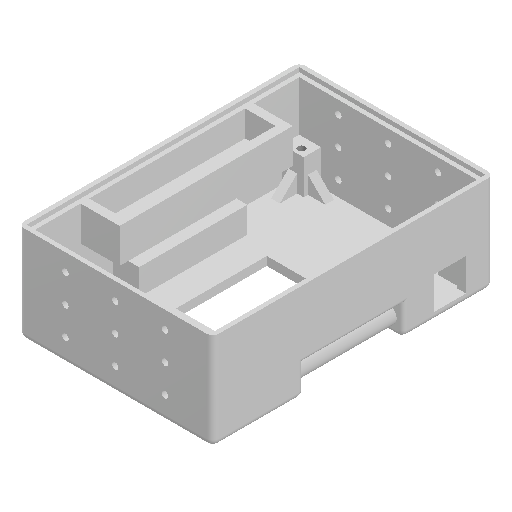
# Autodesk Inventor part: Base
Saved by Autodesk Inventor 2025.2 (Build 292293000, 293)
## iProperties
Created: 2025-10-17
Part Number: Base
Material: ABS Plastic
Document SubType Name: Modeling
Designer: Ricardo
Density: 1.06 g/cm^3
Appearance: Smooth - White
Author: Ricardo
Autodesk Inventor part; units mm, degrees
ref_plane "YZ Plane" through (0, 0, 0) normal (1, 0, 0) x (0, 1, 0)
ref_plane "XZ Plane" through (0, 0, 0) normal (0, 1, 0) x (-1, 0, 0)
ref_plane "XY Plane" through (0, 0, 0) normal (0, 0, 1) x (1, 0, 0)
sketch "Sketch1" plane through (0, 0, 0) normal (0, 1, 0) x (-1, 0, 0)
  line L0 (0, 0) -> (45, 0)
  line L1 (45, 0) -> (45, -65)
  line L2 (45, -65) -> (0, -65)
  line L3 (0, -65) -> (0, 0)
  dimension "d0" = 45
  dimension "d1" = 65
  constraints: 8 end point, 2 parallel, 1 horizontal, 1 perpendicular
  measures "d0" distance of L1.end L2.end
  measures "d1" distance of L0.end L1.end
extrude "Extrusion1" add sketch "Sketch1" against normal blind 3.5
sketch "Sketch2" plane through (0, 0, 0) normal (0, 1, 0) x (1, 0, 0)
  line L0 (-43, 2) -> (-2, 2)
  line L1 (-2, 2) -> (-2, 63)
  line L2 (-2, 63) -> (-43, 63)
  line L3 (-43, 63) -> (-43, 2)
  line L4 (0, 65) -> (-45, 65) projected
  line L5 (-45, 65) -> (-45, 0) projected
  line L6 (-45, 0) -> (0, 0) projected
  line L7 (0, 0) -> (0, 65) projected
  dimension "d4" = 2
  dimension "d5" = 2
  dimension "d6" = 2
  dimension "d7" = 2
  constraints: 8 end point, 2 parallel, 1 horizontal, 1 perpendicular
  measures "d4" distance between parallel lines of L5 L3
  measures "d5" distance between parallel lines of L4 L2
  measures "d6" distance between parallel lines of L7 L1
  measures "d7" distance between parallel lines of L6 L0
extrude "Extrusion2" cut sketch "Sketch2" against normal blind 1.5 contours L3 L2 L1 L0
sketch "Sketch3" plane through (0, -1.5, 0) normal (0, 1, 0) x (1, 0, 0)
  line L0 (-2, 63) -> (-2, 2) projected
  line L1 (-43, 63) -> (-2, 63) projected
  line L2 (-43, 2) -> (-43, 63) projected
  line L3 (-2, 2) -> (-43, 2) projected
  line L4 (-45, 0) -> (0, 0) projected
  line L5 (0, 65) -> (-45, 65) projected
  line L6 (0, 0) -> (0, 65) projected
  line L7 (-45, 65) -> (-45, 0) projected
  line L8 (-30.5, 22) -> (-14.5, 22)
  line L9 (-14.5, 22) -> (-14.5, 43)
  line L10 (-14.5, 43) -> (-30.5, 43)
  line L11 (-30.5, 43) -> (-30.5, 22)
  line L12 (-43, 2) -> (-43, 63) projected
  line L13 (-22.5, 0) -> (-22.5, 65) construction
  line L14 (0, 32.5) -> (-45, 32.5) construction
  dimension "d10" = 16
  dimension "d11" = 21
  constraints: 12 end point, 4 midpoint, 3 parallel, 1 horizontal, 1 perpendicular, 2 other
  measures "d10" distance of L10.end L9.end
  measures "d11" distance of L10.end L8.start
extrude "Extrusion3" cut sketch "Sketch3" against normal blind 3 contours L11 L10 L9 L8
sketch "Sketch4" plane through (0, -1.5, 0) normal (0, 1, 0) x (1, 0, 0)
  line L0 (-30.5, 22) -> (-30.5, 43) construction
  line L1 (-14.5, 43) -> (-14.5, 22) construction
  line L2 (-14.5, 32.5) -> (-30.5, 32.5) construction
  line L3 (-45, 65) -> (0, 65) construction
  line L4 (-22.5, 65) -> (-22.5, 5) construction
  circle A0 centre (-22.5, 12) radius 5.25
  circle A1 centre (-22.5, 12) radius 6
  line L5 (-45, 0) -> (0, 0) projected
  line L6 (-22.5, 12) -> (-30.82, 16.8036) construction
  line L7 (-22.5, 12) -> (-31.5933, 6.75) construction
  line L8 (-27.0466, 14.625) -> (-27.8953, 14.625)
  line L9 (-27.0466, 9.375) -> (-27.8953, 9.375)
  point P0 (-28.3926, 10.8696)
  point P1 (-27.637, 10.9167)
  dimension "d14" = 10.5
  dimension "d15" = 12
  dimension "d181" = 12
  dimension "d200" = 60
  dimension "d201" = 60
  constraints: 12 end point, 6 point on circle, 4 midpoint, 2 centre point, 2 point on line, 1 coincident, 1 horizontal, 1 parallel, 1 vertical
  measures "d14" diameter of A0
  measures "d15" diameter of A1
  measures "d181" distance from line of L5 A0.centre
  measures "d200" angle of L4 L7
  measures "d201" angle of L6 L4
sketch "Sketch6" plane through (0, -1.5, 0) normal (0, 1, 0) x (1, 0, 0)
  line L0 (-14.5, 43) -> (-30.5, 43) projected
  line L1 (-30.5, 43) -> (-30.5, 22) projected
  line L2 (-30.5, 22) -> (-14.5, 22) projected
  line L3 (-14.5, 22) -> (-14.5, 43) projected
  line L4 (-2, 63) -> (-43, 63) projected
  line L5 (-43, 63) -> (-43, 2) projected
  line L6 (-43, 2) -> (-2, 2) projected
  line L7 (-2, 2) -> (-2, 63) projected
  line L8 (-45, 0) -> (-45, 65) projected
  line L9 (-45, 65) -> (0, 65) projected
  line L10 (0, 65) -> (0, 0) projected
  line L11 (0, 0) -> (-45, 0) projected
  line L12 (-43, 2) -> (-43, 63) projected
  line L13 (-43, 63) -> (-38, 63)
  line L14 (-38, 63) -> (-38, 59)
  line L15 (-38, 59) -> (-43, 59)
  line L16 (-43, 59) -> (-43, 63)
  line L17 (-43, 63) -> (-2, 63) projected
  line L18 (-2, 63) -> (-7, 63)
  line L19 (-7, 63) -> (-7, 59)
  line L20 (-7, 59) -> (-2, 59)
  line L21 (-2, 59) -> (-2, 63)
  line L22 (-43, 2) -> (-38, 2)
  line L23 (-38, 2) -> (-38, 6)
  line L24 (-38, 6) -> (-43, 6)
  line L25 (-43, 6) -> (-43, 2)
  line L26 (-2, 2) -> (-7, 2)
  line L27 (-7, 2) -> (-7, 6)
  line L28 (-7, 6) -> (-2, 6)
  line L29 (-2, 6) -> (-2, 2)
  point P0 (-43, 59)
  point P1 (-2, 59)
  point P2 (-2, 6)
  dimension "d30" = 5
  dimension "d31" = 4
  dimension "d32" = 5
  dimension "d33" = 4
  dimension "d34" = 5
  dimension "d35" = 4
  dimension "d36" = 5
  dimension "d37" = 4
  constraints: 32 end point, 8 parallel, 4 horizontal, 4 perpendicular
  measures "d30" distance of L14.end L15.end
  measures "d31" distance of L13.end L14.end
  measures "d32" distance of L20.end L19.end
  measures "d33" distance of L18.end L19.end
  measures "d34" distance of L24.end L23.end
  measures "d35" distance of L22.end L23.end
  measures "d36" distance of L27.end L28.end
  measures "d37" distance of L26.end L27.end
extrude "Extrusion6" add sketch "Sketch6" along normal blind 8 contours L7 L20 L19 L4 | L14 L15 L5 L4 | L7 L6 L27 L28 | L24 L23 L6 L5
sketch "Sketch7" plane through (0, 6.5, 0) normal (0, 1, 0) x (1, 0, 0)
  line L0 (-2, 63) -> (-2, 59) projected
  line L1 (-2, 59) -> (-7, 59) projected
  line L2 (-7, 59) -> (-7, 63) projected
  line L3 (-7, 63) -> (-2, 63) projected
  line L4 (-7, 6) -> (-2, 6) projected
  line L5 (-2, 6) -> (-2, 2) projected
  line L6 (-2, 2) -> (-7, 2) projected
  line L7 (-7, 2) -> (-7, 6) projected
  line L8 (-38, 59) -> (-43, 59) projected
  line L9 (-43, 59) -> (-43, 63) projected
  line L10 (-43, 63) -> (-38, 63) projected
  line L11 (-38, 63) -> (-38, 59) projected
  line L12 (-43, 2) -> (-43, 6) projected
  line L13 (-43, 6) -> (-38, 6) projected
  line L14 (-38, 6) -> (-38, 2) projected
  line L15 (-38, 2) -> (-43, 2) projected
  line L16 (-43, 4) -> (-40, 4) construction
  line L17 (-39.4871, 2) -> (-39.4871, 4.5) construction
  line L18 (-43, 6) -> (-43, 59) projected
  line L19 (-2, 59) -> (-2, 6) projected
  line L20 (0, 0) -> (-45, 0) construction
  line L21 (-22.5, 0) -> (-22.5, 65) construction
  line L22 (-45, 65) -> (0, 65) construction
  point P0 (-5, 60.5)
  point P1 (-5, 4.5)
  point P2 (-40, 60.5)
  dimension "d49" = 3
  dimension "d50" = 2.5
  dimension "d51" = 3
  dimension "d52" = 2.5
  dimension "d53" = 3
  dimension "d54" = 2.5
  dimension "d55" = 2.5
  dimension "d56" = 3
  constraints: 6 end point, 3 midpoint, 1 coincident, 1 horizontal, 1 perpendicular, 1 point on line
  measures "d49" distance of L16.start L16.end
  measures "d50" distance of L17.start L17.end
  measures "d51" distance from line of L5 point (-5, 4.5)
  measures "d52" distance from line of L6 point (-5, 4.5)
  measures "d53" distance from line of L19 point (-5, 60.5)
  measures "d54" distance from line of L3 point (-5, 60.5)
  measures "d55" distance from line of L10 point (-40, 60.5)
  measures "d56" distance from line of L9 point (-40, 60.5)
hole "Hole1" at (-5, 6.5, -60.5) at (-5, 6.5, -4.5) at (-39.4871, 6.5, -4.5) at (-40, 6.5, -60.5) direction (0, -1, 0) diameter 1.7294 depth 3 tip angle 118 thread size "M2x0.25" class "6H" standard "ISO Metric profile"
sketch "Sketch8" plane through (0, 0, 0) normal (0, 1, 0) x (1, 0, 0)
  line L0 (-43, 2) -> (-43, 6) projected
  line L1 (-43, 6) -> (-38, 6) projected
  line L2 (-38, 6) -> (-38, 2) projected
  line L3 (-38, 2) -> (-43, 2) projected
  line L4 (-43, 59) -> (-43, 6) projected
  line L5 (-43, 59) -> (-43, 63) projected
  line L6 (-43, 63) -> (-38, 63) projected
  line L7 (-38, 63) -> (-38, 59) projected
  line L8 (-38, 2) -> (-7, 2) projected
  line L9 (-2, 2) -> (-7, 2) projected
  line L10 (-2, 6) -> (-2, 2) projected
  line L11 (-7, 6) -> (-2, 6) projected
  line L12 (-7, 2) -> (-7, 6) projected
  line L13 (-7, 63) -> (-38, 63) projected
  line L14 (-7, 63) -> (-2, 63) projected
  line L15 (-2, 63) -> (-2, 59) projected
  line L16 (-2, 59) -> (-7, 59) projected
  line L17 (-7, 59) -> (-7, 63) projected
  line L18 (-2, 6) -> (-2, 59) projected
  line L19 (-45, 0) -> (-45, 65) projected
  line L20 (-45, 65) -> (0, 65) projected
  line L21 (0, 65) -> (0, 0) projected
  line L22 (0, 0) -> (-45, 0) projected
  line L23 (-45, 0) -> (0, 0)
  line L24 (0, 0) -> (0, 65)
  line L25 (0, 65) -> (-45, 65)
  line L26 (-45, 65) -> (-45, 0)
  line L27 (-2, 63) -> (-43, 63)
  line L28 (-43, 63) -> (-43, 2)
  line L29 (-43, 2) -> (-2, 2)
  line L30 (-2, 2) -> (-2, 63)
  line L31 (-43, 6) -> (-43, 59) projected
  line L32 (-45, 65) -> (-45, 0) projected
  line L33 (0, 65) -> (-45, 65) projected
  line L34 (-38, 63) -> (-7, 63) projected
  line L35 (-38, 63) -> (-43, 63) projected
  line L36 (0, 0) -> (0, 65) projected
  line L37 (-2, 59) -> (-2, 6) projected
  line L38 (-7, 2) -> (-38, 2) projected
  line L39 (-45, 0) -> (0, 0) projected
  line L40 (-43, 2) -> (-2, 2)
  line L41 (-2, 2) -> (-2, 63)
  line L42 (-2, 63) -> (-43, 63)
  line L43 (-43, 63) -> (-43, 2)
  line L44 (0, 0) -> (-45, 0)
  line L45 (-45, 0) -> (-45, 65)
  line L46 (-45, 65) -> (0, 65)
  line L47 (0, 65) -> (0, 0)
  line L48 (-38, 59) -> (-43, 59) projected
  point P0 (-38.13, 58.5)
  point P1 (-37.5, 3.3857)
  point P2 (-38.5896, 4.5)
  point P3 (-5.5, 3.3968)
  point P4 (-4.3968, 4.5)
  point P5 (-39.1545, 59)
  point P6 (-38, 5.2834)
  point P7 (-38, 59.903)
  point P8 (-2.7165, 59)
  constraints: 32 end point, 8 parallel, 4 horizontal, 4 perpendicular
extrude "Extrusion7" add sketch "Sketch8" along normal blind 18
sketch "Sketch9" plane through (0, 18, 0) normal (0, 1, 0) x (1, 0, 0)
  line L0 (-45, 65) -> (-45, 0) projected
  line L1 (-45, 0) -> (0, 0) projected
  line L2 (0, 0) -> (0, 65) projected
  line L3 (0, 65) -> (-45, 65) projected
  line L4 (-1, 1) -> (-44, 1)
  line L5 (-44, 1) -> (-44, 64)
  line L6 (-44, 64) -> (-1, 64)
  line L7 (-1, 64) -> (-1, 1)
  line L8 (-45, 0) -> (0, 0)
  line L9 (0, 0) -> (0, 65)
  line L10 (0, 65) -> (-45, 65)
  line L11 (-45, 65) -> (-45, 0)
  line L12 (0, 0) -> (-45, 0)
  line L13 (0, 65) -> (0, 0) projected
  line L14 (0, 0) -> (-45, 0) projected
  line L15 (-45, 0) -> (-45, 65) projected
  line L16 (-45, 65) -> (0, 65) projected
  line L17 (-2, 2) -> (-2, 63) projected
  line L18 (-2, 63) -> (-43, 63) projected
  line L19 (-43, 63) -> (-43, 2) projected
  line L20 (-43, 2) -> (-2, 2) projected
  line L21 (-45, 0) -> (0, 0)
  line L22 (0, 0) -> (0, 65)
  line L23 (0, 65) -> (-45, 65)
  line L24 (-45, 65) -> (-45, 0)
  dimension "d57" = 1
  dimension "d58" = 1
  dimension "d59" = 1
  dimension "d60" = 1
  constraints: 26 end point, 7 equal length, 3 horizontal, 3 perpendicular
  measures "d57" distance between parallel lines of L3 L6
  measures "d58" distance between parallel lines of L0 L5
  measures "d59" distance between parallel lines of L1 L4
  measures "d60" distance between parallel lines of L2 L7
extrude "Extrusion8" add sketch "Sketch9" along normal blind 1 contours L3 L2 L1 L0
fillet "Fillet3" radius 1.5 1 edges at (-22.5, -3.5, 0)
fillet "Fillet4" radius 1.5 1 edges at (-22.5, -3.5, -65)
sketch "Sketch10" plane through (-45, 19, -65) normal (-1, 0, 0) x (0, 0, 1)
  line L0 (18, -15.5) -> (12, -15.5) construction
  line L1 (18, -14) -> (12, -14)
  line L2 (12, -17) -> (18, -17)
  arc A0 (18, -17) -> (18, -14) centre (18, -15.5) ccw
  arc A1 (12, -14) -> (12, -17) centre (12, -15.5) ccw
  line L3 (63.5, -22.5) -> (1.5, -22.5) projected
  line L4 (0, -21) -> (0, 0) projected
  point P0 (65, -19)
  point P1 (15, -15.5)
  point P2 (0, -9.5)
  point P3 (0, -6.5)
  dimension "d65" = 6
  dimension "d66" = 3
  dimension "d67" = 5.5
  dimension "d71" = 15
  constraints: 8 end point, 4 point on circle, 4 tangent, 2 centre point, 1 horizontal, 1 midpoint, 1 parallel
  measures "d65" distance of L0.start L0.end
  measures "d66" diameter of A1
  measures "d67" distance between parallel lines of L3 L2
  measures "d71" distance from line of L4 point (15, -15.5)
extrude "Extrusion9" cut sketch "Sketch10" against normal blind 10
sketch "Sketch13" plane through (0, 19, 0) normal (1, 0, 0) x (0, 0, -1)
  line L0 (59, -20.5) -> (6, -20.5) projected
  line L1 (59, -20.5) -> (63, -20.5) projected
  line L2 (63, -20.5) -> (63, -12.5) projected
  line L3 (51, -13) -> (58.5, -13)
  line L4 (58.5, -13) -> (58.5, -20.5)
  line L5 (58.5, -20.5) -> (51, -20.5)
  line L6 (51, -20.5) -> (51, -13)
  line L7 (51, -16.75) -> (58.5, -16.75) construction
  line L8 (54.75, -20.5) -> (54.75, -13) construction
  line L9 (65, 0) -> (65, -21) construction
  point P0 (0, -19)
  dimension "d82" = 7.5
  dimension "d83" = 7.5
  dimension "d84" = 0
  dimension "d86" = 6.5
  constraints: 12 end point, 4 midpoint, 2 parallel, 1 horizontal, 1 perpendicular
  measures "d82" distance of L4.end L5.end
  measures "d83" distance of L3.end L4.end
  measures "d84" distance between parallel lines of L0 L5
  measures "d86" distance between parallel lines of L9 L4
extrude "Extrusion11" cut sketch "Sketch13" against normal blind 10
sketch "Sketch17" plane through (0, -1.5, 0) normal (0, 1, 0) x (1, 0, 0)
  line L0 (-8, 45) -> (0, 45)
  line L1 (0, 45) -> (0, 20)
  line L2 (0, 20) -> (-8, 20)
  line L3 (-8, 20) -> (-8, 45)
  line L4 (0, 65) -> (-45, 65) projected
  line L5 (0, 0) -> (0, 65) projected
  line L6 (-22.5, 65) -> (-22.5, 0) construction
  line L7 (0, 0) -> (-45, 0) construction
  line L8 (-37, 45) -> (-45, 45)
  line L9 (-45, 45) -> (-45, 20)
  line L10 (-45, 20) -> (-37, 20)
  line L11 (-37, 20) -> (-37, 45)
  dimension "d104" = 8
  dimension "d105" = 25
  dimension "d106" = 20
  dimension "d107" = 0
  constraints: 18 end point, 4 symmetric about line, 2 midpoint, 2 parallel, 1 horizontal, 1 perpendicular
  measures "d104" distance of L1.end L2.end
  measures "d105" distance of L2.end L0.start
  measures "d106" distance from line of L4 L0.start
  measures "d107" distance between parallel lines of L5 L1
extrude "Extrusion16" add sketch "Sketch17" along normal blind 6
sketch "Sketch19" plane through (-45, 19, -65) normal (-1, 0, 0) x (0, 0, 1)
  arc A0 (18, -17) -> (18, -14) centre (18, -15.5) ccw projected
  line L0 (18, -14) -> (12, -14) projected
  arc A1 (12, -14) -> (12, -17) centre (12, -15.5) ccw projected
  line L1 (12, -17) -> (18, -17) projected
  arc A2 (0, -21) -> (1.5, -22.5) centre (1.5, -21) ccw projected
  line L2 (0, -21) -> (0, 0) projected
  line L3 (0, 0) -> (65, 0) projected
  line L4 (65, 0) -> (65, -21) projected
  arc A3 (63.5, -22.5) -> (65, -21) centre (63.5, -21) ccw projected
  line L5 (63.5, -22.5) -> (1.5, -22.5) projected
  line L6 (45, -14.5) -> (20, -14.5) projected
  line L7 (20, -14.5) -> (20, -20.5) projected
  line L8 (45, -20.5) -> (45, -14.5) projected
  line L9 (21, -22.5) -> (44, -22.5)
  line L10 (44, -22.5) -> (44, -15.5)
  line L11 (44, -15.5) -> (21, -15.5)
  line L12 (21, -15.5) -> (21, -22.5)
  point P0 (65, -19)
  point P1 (19.5, -7.5)
  point P2 (21, -19)
  point P3 (44, -22.5)
  dimension "d110" = 1
  dimension "d111" = 1
  dimension "d112" = 1
  constraints: 8 end point, 2 parallel, 1 horizontal, 1 midpoint, 1 perpendicular, 1 point on line, 3 other
  measures "d110" distance between parallel lines of L8 L10
extrude "Extrusion17" cut sketch "Sketch19" against normal blind 7 contours L12 L11 L10 L5
sketch "Sketch20" plane through (-45, -3.5, -21) normal (0, 0, -1) x (-1, 0, 0)
  line L0 (0, 7) -> (0, 0) projected
  line L1 (0, 0) -> (-7, 0) projected
  circle A0 centre (-3.5, 3.5) radius 2
  point P0 (-45, 3.5)
  dimension "d115" = 3.5
  dimension "d116" = 3.5
  dimension "d117" = 4
  constraints: 1 centre point, 1 coincident
  measures "d115" distance from line of L0 point (-3.5, 3.5)
  measures "d116" distance from line of L1 point (-3.5, 3.5)
  measures "d117" diameter of A0
extrude "Extrusion18" add sketch "Sketch20" along normal blind 24
sketch "Sketch21" plane through (0, 19, 0) normal (1, 0, 0) x (0, 0, -1)
  line L0 (58.5, -20.5) -> (58.5, -13) projected
  line L1 (58.5, -13) -> (51, -13) projected
  line L2 (51, -13) -> (51, -20.5) projected
  line L3 (51, -20.5) -> (58.5, -20.5) projected
  line L4 (0, 0) -> (65, 0) projected
  line L5 (65, 0) -> (65, -21) projected
  arc A0 (63.5, -22.5) -> (65, -21) centre (63.5, -21) ccw projected
  line L6 (63.5, -22.5) -> (1.5, -22.5) projected
  arc A1 (0, -21) -> (1.5, -22.5) centre (1.5, -21) ccw projected
  line L7 (0, -21) -> (0, 0) projected
  line L8 (44, -15.5) -> (21, -15.5) projected
  line L9 (44, -22.5) -> (44, -15.5) projected
  line L10 (21, -15.5) -> (21, -22.5) projected
  line L11 (21, -22.5) -> (44, -22.5)
  line L12 (44, -22.5) -> (44, -15.5)
  line L13 (44, -15.5) -> (21, -15.5)
  line L14 (21, -15.5) -> (21, -22.5)
  point P0 (0, -19)
  constraints: 8 end point, 2 parallel, 1 horizontal, 1 perpendicular
extrude "Extrusion20" cut sketch "Sketch21" against normal blind 7 contours L10 L8 L9 L6
sketch "Sketch22" plane through (0, -3.5, -44) normal (0, 0, 1) x (1, 0, 0)
  line L0 (0, 7) -> (0, 0) projected
  line L1 (0, 0) -> (-7, 0) projected
  circle A0 centre (-3.5, 3.5) radius 2
  point P0 (0, 3.5)
  dimension "d124" = 3.5
  dimension "d125" = 3.5
  dimension "d126" = 4
  constraints: 1 centre point, 1 coincident
  measures "d124" distance from line of L0 point (-3.5, 3.5)
  measures "d125" distance from line of L1 point (-3.5, 3.5)
  measures "d126" diameter of A0
extrude "Extrusion21" add sketch "Sketch22" along normal blind 24
fillet "Fillet6" radius 1.5 3 edges at (0, -3.0607, -0.4393) (0, 8.5, 0) (0, -3.5, -11.25)
fillet "Fillet9" radius 1 3 edges at (-0.4393, -3.0607, -21) (-4.25, -3.5, -21) (0, 0.75, -21)
fillet "Fillet11" radius 1.5 3 edges at (0, -3.0607, -64.5607) (0, 8.5, -65) (0, -3.5, -53.75)
fillet "Fillet12" radius 1.5 2 edges at (-7, -3.5, -32.5) (-7, -3.5, -20.5)
fillet "Fillet13" radius 1 3 edges at (-0.4393, -3.0607, -44) (0, 0.75, -44) (-5, -3.5, -44)
fillet "Fillet14" radius 1 2 edges at (0, 3.5, -44.5) (0, 3.5, -32)
fillet "Fillet15" radius 1.5 3 edges at (-45, -3.0607, -64.5607) (-45, -3.5, -53.75) (-45, 8.5, -65)
fillet "Fillet16" radius 1.5 3 edges at (-45, -3.0607, -0.4393) (-45, 8.5, 0) (-45, -3.5, -11.25)
sketch "Sketch23" plane through (-43, -1.5, -59) normal (1, 0, 0) x (0, 0, -1)
  line L0 (-46.5, 19.5) -> (-6.5, 19.5)
  line L1 (-6.5, 19.5) -> (-6.5, 11.5)
  line L2 (-6.5, 11.5) -> (-46.5, 11.5)
  line L3 (-46.5, 11.5) -> (-46.5, 19.5)
  line L4 (-57, 19.5) -> (4, 19.5) projected
  point P0 (-59, 1.5)
  point P1 (4, 13.75)
  dimension "d141" = 40
  dimension "d142" = 10.5
  dimension "d151" = 8
  constraints: 8 end point, 2 parallel, 1 horizontal, 1 perpendicular, 1 point on line
  measures "d141" distance of L1.end L2.end
  measures "d142" distance from line of point (4, 13.75) L1
  measures "d151" distance of L0.end L1.end
extrude "Extrusion22" add sketch "Sketch23" along normal blind 9
sketch "Sketch24" plane through (0, 18, 0) normal (0, 1, 0) x (1, 0, 0)
  line L0 (-43, 52.5) -> (-34, 52.5) projected
  line L1 (-34, 52.5) -> (-34, 12.5) projected
  line L2 (-43, 12.5) -> (-34, 12.5) projected
  line L3 (-44, 64) -> (-44, 1) projected
  line L4 (-36, 50.5) -> (-43, 50.5)
  line L5 (-43, 50.5) -> (-43, 14.5)
  line L6 (-43, 14.5) -> (-36, 14.5)
  line L7 (-36, 14.5) -> (-36, 50.5)
  line L8 (-43, 52.5) -> (-43, 12.5) projected
  point P0 (0, 0)
  point P1 (-39.5, 14.5)
  dimension "d145" = 2
  dimension "d146" = 2
  dimension "d147" = 2
  dimension "d148" = 0
  constraints: 8 end point, 2 parallel, 1 horizontal, 1 midpoint, 1 perpendicular
  measures "d145" distance between parallel lines of L1 L7
  measures "d146" distance between parallel lines of L0 L4
  measures "d147" distance from line of L2 point (-39.5, 14.5)
  measures "d148" distance between parallel lines of L8 L5
extrude "Extrusion25" cut sketch "Sketch24" against normal blind 6 contours L4 L7 L6 L5
sketch "Sketch25" plane through (-7, -1.5, -63) normal (-1, 0, 0) x (0, 0, 1)
  line L0 (0, 8) -> (4, 8) projected
  line L1 (4, 0) -> (4, 8) projected
  line L2 (4, 0) -> (0, 0) projected
  line L3 (1, 0) -> (3, 0)
  line L4 (3, 0) -> (3, 4)
  line L5 (3, 4) -> (1, 4)
  line L6 (1, 4) -> (1, 0)
  point P0 (63, 1.5)
  point P1 (3, 0)
  dimension "d157" = 2
  dimension "d158" = 1
  dimension "d159" = 4
  constraints: 8 end point, 2 parallel, 1 horizontal, 1 perpendicular, 1 point on line
  measures "d157" distance of L5.end L4.end
  measures "d158" distance between parallel lines of L1 L4
  measures "d159" distance of L3.end L4.end
extrude "Extrusion26" add sketch "Sketch25" along normal blind 4
sketch "Sketch26" plane through (-7, -1.5, -60) normal (0, 0, 1) x (1, 0, 0)
  line L0 (0, 4) -> (0, 0) construction
  line L1 (0, 4) -> (-4, 4) construction
  line L2 (-4, 0) -> (-4, 4) construction
  line L3 (0, 0) -> (-4, 0) construction
  line L4 (-4, 0) -> (0, 0) construction
  line L5 (0, 4) -> (-4, 0) construction
  line L6 (-4, 0) -> (0, 4)
  line L7 (-4, 0) -> (-4, 4) projected
  line L8 (-4, 4) -> (-4, 0)
  line L9 (-4, 0) -> (0, 4)
  line L10 (-4, 4) -> (0, 4)
  point P0 (7, 1.5)
  constraints: 12 end point, 3 collinear, 1 point on line
extrude "Extrusion27" cut sketch "Sketch26" against normal blind 2
sketch "Sketch27" plane through (-38, -1.5, -59) normal (1, 0, 0) x (0, 0, -1)
  line L0 (0, 8) -> (4, 8) projected
  line L1 (0, 0) -> (0, 8) projected
  line L2 (4, 8) -> (4, 0) projected
  line L3 (4, 0) -> (0, 0) projected
  line L4 (4, 8) -> (4, 0) projected
  line L5 (0, 8) -> (4, 8) projected
  line L6 (0, 0) -> (0, 8) projected
  line L7 (0, 0) -> (0, 8) projected
  line L8 (0, 0) -> (0, 8) projected
  line L9 (0, 0) -> (0, 8) projected
  line L10 (4, 0) -> (0, 0) projected
  line L11 (3, 0) -> (1, 0)
  line L12 (1, 0) -> (1, 4)
  line L13 (1, 4) -> (3, 4)
  line L14 (3, 4) -> (3, 0)
  point P0 (-59, 1.5)
  point P1 (1, 0)
  point P2 (3, 0)
  dimension "d164" = 2
  dimension "d165" = 1
  dimension "d166" = 4
  constraints: 8 end point, 2 parallel, 1 horizontal, 1 perpendicular, 1 point on line
  measures "d164" distance of L12.end L13.end
  measures "d165" distance between parallel lines of L2 L14
  measures "d166" distance of L11.end L12.end
extrude "Extrusion28" add sketch "Sketch27" along normal blind 4 contours L12 L13 L14 L3
sketch "Sketch28" plane through (-38, -1.5, -60) normal (0, 0, 1) x (1, 0, 0)
  line L0 (0, 4) -> (4, 4) projected
  line L1 (4, 4) -> (4, 0) projected
  line L2 (4, 0) -> (0, 0) projected
  line L3 (0, 0) -> (0, 4) projected
  line L4 (0, 4) -> (4, 0)
  line L5 (4, 4) -> (4, 0)
  line L6 (4, 4) -> (0, 4)
  point P0 (38, 1.5)
  constraints: 6 end point, 1 collinear
extrude "Extrusion29" cut sketch "Sketch28" against normal blind 2 contours L0 L1 L4
sketch "Sketch29" plane through (-43, -1.5, -59) normal (0, 0, 1) x (1, 0, 0)
  line L0 (5, 0) -> (0, 0) projected
  line L1 (5, 0) -> (5, 8) projected
  line L2 (0, 8) -> (5, 8) projected
  line L3 (0, 0) -> (0, 8) projected
  line L4 (5, 0) -> (0, 0) projected
  line L5 (1.5, 0) -> (3.5, 0)
  line L6 (3.5, 0) -> (3.5, 4)
  line L7 (3.5, 4) -> (1.5, 4)
  line L8 (1.5, 4) -> (1.5, 0)
  point P0 (43, 1.5)
  point P1 (1.5, 0)
  point P2 (3.5, 0)
  dimension "d171" = 2
  dimension "d172" = 1.5
  dimension "d173" = 4
  constraints: 8 end point, 2 parallel, 1 horizontal, 1 perpendicular, 1 point on line
  measures "d171" distance of L7.end L6.end
  measures "d172" distance between parallel lines of L1 L6
  measures "d173" distance of L5.end L6.end
extrude "Extrusion30" add sketch "Sketch29" along normal blind 4 contours L0 L8 L7 L6
sketch "Sketch30" plane through (-39.5, -1.5, -59) normal (1, 0, 0) x (0, 0, -1)
  line L0 (0, 4) -> (-4, 4) projected
  line L1 (-4, 0) -> (-4, 4) projected
  line L2 (0, 0) -> (-4, 0) projected
  line L3 (0, 4) -> (0, 0) projected
  line L4 (-4, 0) -> (0, 4)
  line L5 (0, 4) -> (-4, 4)
  line L6 (0, 0) -> (0, 8) projected
  line L7 (-4, 0) -> (-4, 4)
  point P0 (-59, 1.5)
  constraints: 6 end point, 1 collinear, 1 perpendicular
extrude "Extrusion31" cut sketch "Sketch30" against normal blind 2 contours L4 L1 L0
sketch "Sketch31" plane through (-2, -1.5, -6) normal (0, 0, -1) x (-1, 0, 0)
  line L0 (1.5, 4) -> (3.5, 4)
  line L1 (3.5, 4) -> (3.5, 0)
  line L2 (3.5, 0) -> (1.5, 0)
  line L3 (1.5, 0) -> (1.5, 4)
  line L4 (5, 0) -> (5, 8) projected
  line L5 (5, 0) -> (0, 0) projected
  point P0 (-2, 1.5)
  dimension "d178" = 2
  dimension "d179" = 1.5
  dimension "d180" = 4
  constraints: 8 end point, 2 parallel, 1 horizontal, 1 perpendicular, 1 point on line
  measures "d178" distance of L1.end L2.end
  measures "d179" distance between parallel lines of L4 L1
  measures "d180" distance of L0.end L1.end
extrude "Extrusion32" add sketch "Sketch31" along normal blind 4
sketch "Sketch32" plane through (-5.5, -1.5, -6) normal (-1, 0, 0) x (0, 0, 1)
  line L0 (0, 4) -> (0, 0) projected
  line L1 (0, 4) -> (-4, 4) projected
  line L2 (-4, 0) -> (-4, 4) projected
  line L3 (0, 0) -> (-4, 0) projected
  line L4 (-4, 0) -> (0, 4)
  line L5 (0, 4) -> (-4, 4)
  line L6 (-4, 4) -> (-4, 0)
  point P0 (6, 1.5)
  constraints: 6 end point, 2 collinear
extrude "Extrusion33" cut sketch "Sketch32" against normal blind 2 contours L4 L2 L1
sketch "Sketch33" plane through (-7, -1.5, -6) normal (-1, 0, 0) x (0, 0, 1)
  line L0 (4, 0) -> (0, 0) projected
  line L1 (4, 8) -> (4, 0) projected
  line L2 (0, 8) -> (4, 8) projected
  line L3 (0, 0) -> (0, 8) projected
  line L4 (1, 4) -> (3, 4)
  line L5 (3, 4) -> (3, 0)
  line L6 (3, 0) -> (1, 0)
  line L7 (1, 0) -> (1, 4)
  point P0 (6, 1.5)
  point P1 (2, 0)
  point P2 (1, 0)
  point P3 (3, 0)
  dimension "d186" = 2
  dimension "d187" = 1
  dimension "d188" = 4
  constraints: 8 end point, 2 midpoint, 2 parallel, 1 horizontal, 1 perpendicular
  measures "d186" distance of L5.end L6.end
  measures "d187" distance between parallel lines of L3 L7
  measures "d188" distance of L6.end L4.start
extrude "Extrusion34" add sketch "Sketch33" along normal blind 4 contours L0 L7 L4 L5
sketch "Sketch34" plane through (-7, -1.5, -5) normal (0, 0, -1) x (-1, 0, 0)
  line L0 (0, 0) -> (0, 4) projected
  line L1 (4, 0) -> (0, 0) projected
  line L2 (4, 4) -> (4, 0) projected
  line L3 (0, 4) -> (4, 4) projected
  line L4 (0, 4) -> (4, 0)
  line L5 (4, 4) -> (4, 0) projected
  line L6 (4, 4) -> (0, 4)
  point P0 (-7, 1.5)
  constraints: 4 end point
extrude "Extrusion35" cut sketch "Sketch34" against normal blind 2 contours L3 L2 L4
sketch "Sketch35" plane through (-38, -1.5, -2) normal (1, 0, 0) x (0, 0, -1)
  line L0 (4, 0) -> (0, 0) projected
  line L1 (4, 0) -> (4, 8) projected
  line L2 (0, 8) -> (4, 8) projected
  line L3 (0, 0) -> (0, 8) projected
  line L4 (3, 4) -> (1, 4)
  line L5 (1, 4) -> (1, 0)
  line L6 (1, 0) -> (3, 0)
  line L7 (3, 0) -> (3, 4)
  line L8 (4, 0) -> (0, 0) projected
  point P0 (-2, 1.5)
  point P1 (3, 0)
  dimension "d193" = 2
  dimension "d194" = 1
  dimension "d195" = 4
  constraints: 8 end point, 2 parallel, 1 horizontal, 1 perpendicular, 1 point on line
  measures "d193" distance of L6.end L5.end
  measures "d194" distance between parallel lines of L1 L7
  measures "d195" distance of L6.end L4.start
extrude "Extrusion36" add sketch "Sketch35" along normal blind 4 contours L0 L5 L4 L7
sketch "Sketch36" plane through (-38, -1.5, -5) normal (0, 0, -1) x (-1, 0, 0)
  line L0 (0, 4) -> (0, 0) projected
  line L1 (0, 4) -> (-4, 4) projected
  line L2 (-4, 0) -> (-4, 4) projected
  line L3 (0, 0) -> (-4, 0) projected
  line L4 (0, 4) -> (-4, 4) projected
  line L5 (-4, 0) -> (-4, 4)
  line L6 (-4, 4) -> (-4, 0)
  line L7 (0, 4) -> (-4, 4)
  line L8 (0, 4) -> (-4, 0)
  line L9 (-4, 0) -> (-4, 4) projected
  line L10 (-4, 4) -> (0, 4)
  point P0 (-38, 1.5)
  constraints: 10 end point, 2 perpendicular, 1 vertical
extrude "Extrusion37" cut sketch "Sketch36" against normal blind 2 contours L8 L2 L1
extrude "Extrusion38" add sketch "Sketch4" along normal blind 3 contours A0 L8 A1 L9 picked at (-16.8588, 12.8966)
fillet "Fillet18" radius 0.5 1 edges at (-16.5, -1.5, -12)
sketch "Sketch37" plane through (-1.5, -2, 0) normal (0, 0, 1) x (1, 0, 0)
  line L0 (-43.5, 21) -> (-43.5, 0) projected
  line L1 (1.5, 0) -> (1.5, 21) projected
  line L2 (-42, -1.5) -> (0, -1.5) projected
  arc A0 (0, -1.5) -> (1.5, 0) centre (0, 0) ccw projected
  arc A1 (-43.5, 0) -> (-42, -1.5) centre (-42, 0) ccw projected
  line L3 (1.5, 10.5) -> (-43.5, 10.5) construction
  line L4 (-21, -1.5) -> (-21, 26.25) construction
  circle A2 centre (-21, 10.5) radius 0.75
  circle A3 centre (-32.5, 17) radius 0.75
  circle A4 centre (-32.5, 4) radius 0.75
  circle A5 centre (-32.5, 10.5) radius 0.75
  circle A6 centre (-21, 17) radius 0.75
  circle A7 centre (-21, 4) radius 0.75
  line L5 (-42, 21) -> (0, 21) projected
  circle A8 centre (-9.5, 17) radius 0.75
  circle A9 centre (-9.5, 4) radius 0.75
  circle A10 centre (-9.5, 10.5) radius 0.75
  point P0 (1.5, 2)
  dimension "d205" = 1.5
  dimension "d206" = 1.5
  dimension "d207" = 1.5
  dimension "d208" = 1.5
  dimension "d209" = 1.5
  dimension "d210" = 1.5
  dimension "d211" = 11
  dimension "d214" = 6.5
  dimension "d215" = 6.5
  constraints: 9 centre point, 4 end point, 4 midpoint, 4 point on line, 3 symmetric about line, 2 horizontal alignment, 2 vertical alignment, 1 vertical, 3 other
  measures "d205" diameter of A2
  measures "d206" diameter of A3
  measures "d207" diameter of A4
  measures "d208" diameter of A5
  measures "d209" diameter of A6
  measures "d210" diameter of A7
  measures "d211" distance from line of L0 A3.centre
  measures "d214" distance of A3.centre A5.centre
  measures "d215" distance of A4.centre A5.centre
extrude "Extrusion39" cut sketch "Sketch37" against normal blind 5
sketch "Sketch38" plane through (-1.5, -2, -65) normal (0, 0, -1) x (-1, 0, 0)
  line L0 (0, 21) -> (42, 21) projected
  line L1 (42, 0) -> (42, 21) projected
  line L2 (42, 0) -> (0, 0) projected
  line L3 (0, 0) -> (0, 21) projected
  line L4 (0, 21) -> (42, 21) projected
  line L5 (42, 0) -> (42, 21) projected
  line L6 (42, 0) -> (0, 0) projected
  line L7 (0, 0) -> (0, 21) projected
  circle A0 centre (21, 17) radius 0.75 projected
  circle A1 centre (32.5, 4) radius 0.75 projected
  circle A2 centre (9.5, 17) radius 0.75 projected
  circle A3 centre (9.5, 10.5) radius 0.75 projected
  circle A4 centre (21, 4) radius 0.75 projected
  circle A5 centre (32.5, 10.5) radius 0.75 projected
  circle A6 centre (21, 17) radius 0.75 projected
  circle A7 centre (9.5, 4) radius 0.75 projected
  circle A8 centre (21, 10.5) radius 0.75 projected
  circle A9 centre (32.5, 17) radius 0.75 projected
  line L8 (5.5, 8.5) -> (5.5, 0.5) projected
  line L9 (5.5, 0.5) -> (36.5, 0.5) projected
  line L10 (36.5, 0.5) -> (36.5, 8.5) projected
  line L11 (41.5, 8.5) -> (36.5, 8.5) projected
  line L12 (41.5, 8.5) -> (41.5, 20) projected
  line L13 (0.5, 20) -> (41.5, 20) projected
  line L14 (0.5, 8.5) -> (0.5, 20) projected
  line L15 (5.5, 8.5) -> (0.5, 8.5) projected
  line L16 (-1.5, 21) -> (-1.5, 0) projected
  line L17 (43.5, 0) -> (43.5, 21) projected
  line L18 (0, -1.5) -> (42, -1.5) projected
  line L19 (0, 21) -> (42, 21) projected
  circle A10 centre (9.5, 17) radius 0.75
  circle A11 centre (9.5, 10.5) radius 0.75
  circle A12 centre (9.5, 4) radius 0.75
  circle A13 centre (21, 17) radius 0.75
  circle A14 centre (21, 10.5) radius 0.75
  circle A15 centre (21, 4) radius 0.75
  line L20 (29, -1.5) -> (13, -1.5) construction
  line L21 (21, -1.5) -> (21, 21) construction
  circle A16 centre (32.5, 17) radius 0.75
  circle A17 centre (32.5, 10.5) radius 0.75
  circle A18 centre (32.5, 4) radius 0.75
  point P0 (-1.5, 2)
  constraints: 9 centre point, 6 coincident, 5 concentric, 3 symmetric about line, 2 end point, 2 midpoint, 3 other
extrude "Extrusion40" cut sketch "Sketch38" against normal blind 10 contours A0 | A1 | A2 | A3 | A4 | A5 | A7 | A8 | A9
sketch "Sketch42" plane through (-43, -1.5, -6) normal (1, 0, 0) x (0, 0, -1)
  line L0 (41, 6.5) -> (47, 6.5) projected
  line L1 (47, 3.5) -> (41, 3.5) projected
  arc A0 (41, 6.5) -> (41, 3.5) centre (41, 5) ccw projected
  line L2 (47, 3.5) -> (41, 3.5) projected
  arc A1 (41, 6.5) -> (41, 3.5) centre (41, 5) ccw projected
  line L3 (41, 6.5) -> (47, 6.5) projected
  arc A2 (47, 3.5) -> (47, 6.5) centre (47, 5) ccw projected
  line L4 (46.5, 19.5) -> (46.5, 11.5) projected
  line L5 (46.5, 11.5) -> (6.5, 11.5) projected
  line L6 (6.5, 11.5) -> (6.5, 19.5) projected
  line L7 (-4, 19.5) -> (6.5, 19.5) projected
  line L8 (-4, 8) -> (-4, 19.5) projected
  line L9 (0, 8) -> (-4, 8) projected
  line L10 (0, 8) -> (0, 0) projected
  line L11 (0, 0) -> (14, 0) projected
  line L12 (14, 0) -> (14, 6) projected
  line L13 (14, 6) -> (39, 6) projected
  line L14 (39, 6) -> (39, 0) projected
  line L15 (39, 0) -> (53, 0) projected
  line L16 (53, 0) -> (53, 8) projected
  line L17 (57, 8) -> (53, 8) projected
  line L18 (57, 8) -> (57, 19.5) projected
  line L19 (46.5, 19.5) -> (57, 19.5) projected
  line L20 (41, 5) -> (47, 5) construction
  line L21 (41, 3.5) -> (47, 3.5)
  line L22 (47, 6.5) -> (41, 6.5)
  arc A3 (41, 6.5) -> (41, 3.5) centre (41, 5) ccw
  arc A4 (47, 3.5) -> (47, 6.5) centre (47, 5) ccw
  point P0 (-6, 1.5)
  point P1 (44, 5)
  constraints: 8 end point, 4 point on circle, 4 tangent, 2 centre point, 1 concentric, 1 horizontal, 1 midpoint, 1 parallel
extrude "Extrusion41" cut sketch "Sketch42" against normal blind 10 draft 14 contours L0 A2 L1 A0
body "Solid1"
